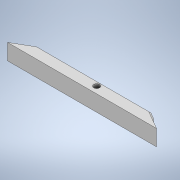
# Autodesk Inventor part: parallel_bar_long_hole_v1
Saved by Autodesk Inventor 2022 (Build 260153000, 153)
## iProperties
Created: 2022-06-04
Part Number: parallel_bar_long_hole_v1
Material: Generic
Document SubType Name: Modeling
Designer: kylem
Density: 1 g/cm^3
Appearance: Default
Author: kylem
Autodesk Inventor part; units mm, degrees
ref_plane "YZ Plane" through (0, 0, 0) normal (1, 0, 0) x (0, 1, 0)
ref_plane "XZ Plane" through (0, 0, 0) normal (0, 1, 0) x (-1, 0, 0)
ref_plane "XY Plane" through (0, 0, 0) normal (0, 0, 1) x (1, 0, 0)
sketch "Sketch1" plane through (0, 0, 0) normal (0, 1, 0) x (-1, 0, 0)
  line L0 (0, 0) -> (56, 0)
  line L1 (56, 0) -> (54.5, 0)
  line L2 (56, 0) -> (21.359, -20)
  line L3 (56, 0) -> (96, 0) construction
  line L4 (28, 0) -> (28, 5.9969)
  line L5 (0, 0) -> (34.641, -20)
  line L6 (28, 0) -> (28, -6)
  line L7 (28, -6) -> (78, -6)
  line L8 (28, -6) -> (-22, -6)
  line L9 (56, 0) -> (53.4019, -1.5)
  line L10 (53.4019, -1.5) -> (39.2598, -15.6421)
  line L11 (53.4019, -1.5) -> (73.4019, -1.5) construction
  line L12 (2.5981, -1.5) -> (16.7402, -15.6421)
  point P0 (48.9019, -6)
  point P1 (7.0981, -6)
  dimension "d0" = 56
  dimension "d3" = 40
  dimension "d4" = 150
  dimension "d5" = 6
  dimension "d6" = 50
  dimension "d7" = 50
  dimension "d8" = 3
  dimension "d9" = 20
  dimension "d10" = 135
  constraints: 26 end point, 5 horizontal, 3 symmetric about line, 2 equal length, 2 vertical, 1 midpoint, 1 perpendicular, 1 point on line
  measures "d0" distance of L0.start L0.end
  measures "d3" distance of L0.end L2.end
  measures "d4" angle of L2 L3
  measures "d5" distance of L4.start L6.end
  measures "d6" distance of L6.end L7.end
  measures "d7" distance of L6.end L8.end
  measures "d8" distance of L0.end L9.end
  measures "d9" distance of L9.end L10.end
  measures "d10" angle of L10 L11
extrude "Extrusion1" add sketch "Sketch1" along normal blind 6 contours L0 L6 L8 L5 | L0 L2 L7 L6 | L5 L8 L12 | L2 L10 L7
chamfer "Chamfer1" distance 2 angle 45 6 edges at (-48.9019, 3, -6) (-51.1519, 6, -3.75) (-51.1519, 0, -3.75) (-4.8481, 0, -3.75) (-7.0981, 3, -6) (-4.8481, 6, -3.75)
chamfer "Chamfer2" distance 2 angle 45 4 edges at (-37.0367, 0, -6) (-18.9633, 0, -6) (-37.0367, 6, -6) (-18.9633, 6, -6)
sketch "Sketch2" plane through (0, 6, 0) normal (0, 1, 0) x (1, 0, 0)
  line L0 (0, 0) -> (-6.9282, 4) projected
  line L1 (0, 0) -> (-25, 0)
  line L2 (-56, 0) -> (0, 0) projected
  line L3 (-25, 0) -> (-25, 2.5)
  line L4 (-25, 0) -> (-22.5, 0) construction
  circle A0 centre (-25, 2.5) radius 1.1
  dimension "d19" = 25
  dimension "d20" = 2.5
  dimension "d21" = 90
  dimension "d22" = 2.2
  constraints: 6 end point, 2 perpendicular, 1 centre point, 1 coincident, 1 horizontal, 1 point on line
  measures "d19" distance of L0.start L1.end
  measures "d20" distance of L1.end L3.end
  measures "d21" angle of L4 L3
  measures "d22" diameter of A0
extrude "Extrusion2" cut sketch "Sketch2" along normal mid plane 50
body "Solid1"
